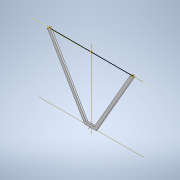
# Autodesk Inventor part: Braccetto
Saved by Autodesk Inventor 2021 (Build 250183000, 183)
## iProperties
Created: 2021-05-04
Part Number: Braccetto
Material: Generic
Document SubType Name: Modeling
Designer: andre
Density: 1 g/cm^3
Appearance: Default
Author: andre
Autodesk Inventor part; units mm, degrees
ref_plane "YZ Plane" through (0, 0, 0) normal (1, 0, 0) x (0, 1, 0)
ref_plane "XZ Plane" through (0, 0, 0) normal (0, 1, 0) x (-1, 0, 0)
sketch "Sketch1" plane through (0, 0, 0) normal (0, 0, 1) x (1, 0, 0)
  line L0 (0, 10) -> (-14.2265, 10)
  line L1 (-14.2265, 10) -> (-138.453, 225.1666)
  line L2 (-138.453, 225.1666) -> (-150, 225.1666)
  line L3 (-150, 225.1666) -> (-20, 0)
  line L4 (-20, 0) -> (0, 0)
  line L5 (0, 0) -> (0, 10)
  dimension "d0" = 260
  dimension "d1" = 30
  dimension "d2" = 10
  dimension "d3" = 10
  dimension "d4" = 20
  constraints: 12 end point, 3 parallel, 1 horizontal, 1 perpendicular
  measures "d0" distance of L2.end L3.end
  measures "d1" angle of L5 L1
  measures "d2" distance of L4.end L0.start
  measures "d3" distance between parallel lines of L3 L1
  measures "d4" distance of L3.end L4.end
extrude "Extrusion1" add sketch "Sketch1" along normal mid plane 5
mirror "Mirror1" about plane through (0, 0, 0) normal (1, 0, 0) of "Extrusion1"
ref_plane "Work Plane1" through (138.453, 225.1666, 2.5) normal (0, -1, 0) x (0, 0, -1)
sketch "Sketch2" plane through (138.453, 225.1666, 2.5) normal (0, -1, 0) x (0, 0, -1)
  line L0 (2.5, -348.453) -> (2.5, 71.547) construction
  line L1 (5, 0) -> (0, 0) construction
  line L2 (5, 11.547) -> (0, 11.547) construction
  line L3 (0, 0) -> (0, 11.547) construction
  line L4 (5, 11.547) -> (5, 0) construction
  line L5 (2.5, 11.547) -> (2.5, 0) construction
  line L6 (5, -276.906) -> (0, -276.906) construction
  line L7 (0, -276.906) -> (0, -288.453) construction
  line L8 (5, -288.453) -> (0, -288.453) construction
  line L9 (5, -288.453) -> (5, -276.906) construction
  line L10 (2.5, -276.906) -> (2.5, -288.453) construction
  line L11 (2.5, 5.7735) -> (2.5, -282.6795)
  line L12 (0, -288.453) -> (0, -158.453) construction
  point P0 (2.5, -138.453)
  constraints: 7 midpoint, 6 end point, 1 parallel, 1 point on line
sketch "Sketch3" plane through (-20, 0, -2.5) normal (0, -1, 0) x (1, 0, 0)
  point P0 (20, 2.5)
  point P1 (20, 2.5)
  constraints: 1 coincident
body "Solid1"
